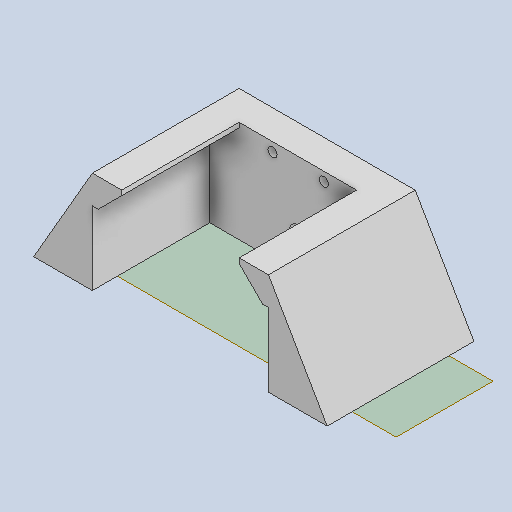
# Autodesk Inventor part: Wheel_well
Saved by Autodesk Inventor 2024 (Build 280153000, 153)
## iProperties
Created: 2025-06-20
Part Number: Wheel_well
Material: Generic
Document SubType Name: Modeling
Designer: Aidan
Density: 1 g/cm^3
Appearance: Default
Author: Aidan
Autodesk Inventor part; units mm, degrees
ref_plane "YZ Plane" through (0, 0, 0) normal (1, 0, 0) x (0, 1, 0)
ref_plane "XZ Plane" through (0, 0, 0) normal (0, 1, 0) x (-1, 0, 0)
ref_plane "XY Plane" through (0, 0, 0) normal (0, 0, 1) x (1, 0, 0)
sketch "Sketch1" plane through (0, 0, 0) normal (0, 0, 1) x (1, 0, 0)
  line L0 (0, 0) -> (100, 0)
  line L1 (0, 0) -> (20, 34.641)
  line L2 (0, 0) -> (40, 0) construction
  line L3 (100, 0) -> (80, 34.641)
  line L4 (100, 0) -> (140, 0) construction
  line L5 (20, 34.641) -> (80, 34.641)
  dimension "d0" = 100
  dimension "d1" = 40
  dimension "d2" = 60
  dimension "d3" = 40
  dimension "d4" = 120
  constraints: 12 end point, 3 horizontal, 2 equal length
  measures "d0" distance of L0.start L0.end
  measures "d1" distance of L0.start L1.end
  measures "d2" angle of L2 L1
  measures "d3" distance of L0.end L3.end
  measures "d4" angle of L4 L3
extrude "Extrusion1" add sketch "Sketch1" along normal blind 30
sketch "Sketch2" plane through (0, 0, 30) normal (0, 0, 1) x (1, 0, 0)
  line L0 (0, 0) -> (100, 0) projected
  line L1 (20, 0) -> (80, 0)
  line L2 (80, 0) -> (80, 25)
  line L3 (80, 25) -> (20, 25)
  line L4 (20, 25) -> (20, 0)
  dimension "d7" = 60
  dimension "d8" = 25
  dimension "d9" = 20
  constraints: 8 end point, 2 parallel, 1 horizontal, 1 perpendicular, 1 point on line
  measures "d7" distance of L3.end L2.end
  measures "d8" distance of L2.end L1.end
  measures "d9" distance from line of L0.start L4
extrude "Extrusion2" cut sketch "Sketch2" against normal blind 20
ref_plane "Work Plane1" through (0, -10, 0) normal (0, -1, 0) x (1, 0, 0)
sketch "Sketch4" plane through (20, 34.641, 0) normal (0, 1, 0) x (1, 0, 0)
  line L0 (60, -10) -> (0, -10) projected
  line L1 (10, -10) -> (50, -10)
  line L2 (50, -10) -> (50, -35)
  line L3 (50, -35) -> (10, -35)
  line L4 (10, -35) -> (10, -10)
  point P0 (-20, 0)
  point P1 (30, -10)
  point P2 (50, -10)
  dimension "d19" = 40
  dimension "d20" = 25
  dimension "d21" = 20
  constraints: 8 end point, 2 parallel, 1 horizontal, 1 midpoint, 1 perpendicular, 1 point on line
  measures "d19" distance of L2.end L3.end
  measures "d20" distance of L1.end L2.end
  measures "d21" distance from line of L4 point (30, -10)
extrude "Extrusion4" cut sketch "Sketch4" against normal through all
chamfer "Chamfer1" distance 8 angle 45 1 edges at (30, 25, 20)
chamfer "Chamfer2" distance 8 angle 45 1 edges at (70, 25, 20)
sketch "Sketch6" plane through (0, 0, 30) normal (0, 0, 1) x (1, 0, 0)
  line L0 (30, 33) -> (22, 25) projected
  line L1 (30, 33) -> (30, 34.641) projected
  line L2 (30, 34.641) -> (20, 34.641) projected
  line L3 (20, 34.641) -> (0, 0) projected
  line L4 (0, 0) -> (20, 0) projected
  line L5 (20, 0) -> (20, 25) projected
  line L6 (20, 25) -> (22, 25) projected
  line L7 (78, 25) -> (70, 33) projected
  line L8 (78, 25) -> (80, 25) projected
  line L9 (80, 25) -> (80, 0) projected
  line L10 (80, 0) -> (100, 0) projected
  line L11 (100, 0) -> (80, 34.641) projected
  line L12 (80, 34.641) -> (70, 34.641) projected
  line L13 (70, 34.641) -> (70, 33) projected
extrude "Extrusion6" add sketch "Sketch6" along normal blind 20
sketch "Sketch8" plane through (0, 0, 0) normal (0, 0, -1) x (-1, 0, 0)
  line L0 (-39.0839, 36.891) -> (-43.0739, 36.891) projected
  line L1 (-43.0739, 48.241) -> (-43.0739, 36.891) projected
  line L2 (-57.1939, 48.241) -> (-43.0739, 48.241) projected
  line L3 (-57.1939, 48.241) -> (-57.1939, 36.891) projected
  line L4 (-57.1939, 36.891) -> (-61.1839, 36.891) projected
  line L5 (-61.1839, 36.891) -> (-61.1839, 5.041) projected
  line L6 (-56.3339, 0.191) -> (-43.9339, 0.191) projected
  line L7 (-39.0839, 5.041) -> (-39.0839, 36.891) projected
  line L8 (-52.9432, 43.5972) -> (-47.3245, 43.5972) projected
  line L9 (-52.9432, 43.5972) -> (-52.9432, 44.1479) projected
  line L10 (-52.4839, 44.6341) -> (-52.9432, 44.1479) projected
  line L11 (-52.4839, 44.6341) -> (-47.7839, 44.6341) projected
  line L12 (-47.3245, 44.1479) -> (-47.7839, 44.6341) projected
  line L13 (-47.3245, 44.1479) -> (-47.3245, 43.5972) projected
  circle A0 centre (-58.8839, 31.541) radius 1.575
  circle A1 centre (-41.3839, 31.541) radius 1.575
  circle A2 centre (-50.1339, 11.541) radius 2.75
  circle A3 centre (-50.1339, 11.541) radius 2.95
  arc A4 (-61.1839, 5.041) -> (-56.3339, 0.191) centre (-56.3339, 5.041) ccw projected
  arc A5 (-43.9339, 0.191) -> (-39.0839, 5.041) centre (-43.9339, 5.041) ccw projected
  circle A6 centre (-50.1339, 11.541) radius 2.75 projected
  circle A7 centre (-41.6839, 2.741) radius 0.75 projected
  circle A8 centre (-58.5839, 2.741) radius 0.75 projected
  circle A9 centre (-40.7939, 35.041) radius 1 projected
  circle A10 centre (-59.4739, 35.041) radius 1 projected
  circle A11 centre (-58.8839, 31.541) radius 1.575 projected
  circle A12 centre (-41.3839, 31.541) radius 1.575 projected
  point P0 (0, 0)
  constraints: 4 centre point, 3 concentric, 1 coincident
extrude "Extrusion8" cut sketch "Sketch8" against normal up to surface (10 mm away) contours A0 | A1 | A2 | A3
body "Solid1"
